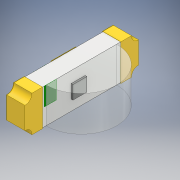
# Autodesk Inventor part: LED 3216 RA
Saved by Autodesk Inventor 2018 (Build 220112000, 112)
## iProperties
Created: 2018-02-20
Part Number: LED 3216 RA
Material: Generic
Document SubType Name: Modeling
Designer: danil
Density: 1 g/cm^3
Appearance: Generic
Author: danil
Autodesk Inventor part; units mm, degrees
ref_plane "YZ Plane" through (0, 0, 0) normal (1, 0, 0) x (0, 1, 0)
ref_plane "XZ Plane" through (0, 0, 0) normal (0, 1, 0) x (-1, 0, 0)
ref_plane "XY Plane" through (0, 0, 0) normal (0, 0, 1) x (1, 0, 0)
sketch "Sketch1" plane through (0, 0, 0) normal (0, 0, 1) x (1, 0, 0)
  arc A0 (0, -1) -> (0, 1) centre (0, 0) ccw
  line L0 (0, 0) -> (0, 1) construction
  line L1 (0, 0) -> (1, 0) construction
  line L2 (0, 0) -> (0, -1) construction
  line L3 (0, 1) -> (0, -1)
  dimension "d0" = 1
  dimension "d1" = 90
  dimension "d2" = 180
  constraints: 8 end point, 2 point on circle, 1 centre point, 1 coincident, 1 horizontal, 1 perpendicular
  measures "d0" radius of A0
  measures "d1" angle of L1 L0
  measures "d2" angle of L2 L0
extrude "Extrusion1" add sketch "Sketch1" along normal blind 1
sketch "Sketch2" plane through (0, -1, 0) normal (-1, 0, 0) x (0, 0, 1)
  line L0 (0, 2.6) -> (1, 2.6)
  line L1 (1, 2.6) -> (1, -0.6)
  line L2 (1, -0.6) -> (0, -0.6)
  line L3 (0, -0.6) -> (0, 2.6)
  line L4 (0, 2) -> (0, 0) projected
  line L5 (1, 2) -> (1, 0) projected
  arc A0 (0, 2.4) -> (0.2, 2.6) centre (0, 2.6) ccw
  arc A1 (0.8, 2.6) -> (1, 2.4) centre (1, 2.6) ccw
  arc A2 (1, -0.4) -> (0.8, -0.6) centre (1, -0.6) ccw
  arc A3 (0.2, -0.6) -> (0, -0.4) centre (0, -0.6) ccw
  point P0 (0, 1)
  point P1 (1, 1)
  point P2 (1, 1)
  dimension "d5" = 3.2
  dimension "d6" = 0.2
  constraints: 8 end point, 8 point on circle, 8 point on line, 5 coincident, 4 centre point, 3 equal radius, 2 collinear, 2 midpoint, 2 parallel, 1 horizontal, 1 perpendicular
  measures "d5" distance of L2.end L0.start
  measures "d6" radius of A0
extrude "Extrusion2" add sketch "Sketch2" along normal blind 0.5 separate body contours L0 A1 L1 A2 L2 A3 L3 A0
sketch "Sketch3" plane through (-0.5, -1, 0) normal (-1, 0, 0) x (0, 0, 1)
  line L0 (0, 2.4) -> (0, -0.4) construction
  arc A0 (0.2, -0.6) -> (0, -0.4) centre (0, -0.6) ccw projected
  line L1 (0.2, -0.6) -> (0.8, -0.6) projected
  arc A1 (1, -0.4) -> (0.8, -0.6) centre (1, -0.6) ccw projected
  line L2 (1, -0.4) -> (1, 2.4) construction
  arc A2 (0.8, 2.6) -> (1, 2.4) centre (1, 2.6) ccw projected
  line L3 (0.8, 2.6) -> (0.2, 2.6) projected
  arc A3 (0, 2.4) -> (0.2, 2.6) centre (0, 2.6) ccw projected
  line L4 (1.01, 2.4103) -> (1.01, -0.4103)
  arc A4 (1.01, -0.4103) -> (0.8103, -0.61) centre (1, -0.6) ccw
  line L5 (0.8103, -0.61) -> (0.1897, -0.61)
  arc A5 (0.1897, -0.61) -> (-0.01, -0.4103) centre (0, -0.6) ccw
  line L6 (-0.01, -0.4103) -> (-0.01, 2.4103)
  arc A6 (-0.01, 2.4103) -> (0.1897, 2.61) centre (0, 2.6) ccw
  line L7 (0.1897, 2.61) -> (0.8103, 2.61)
  arc A7 (0.8103, 2.61) -> (1.01, 2.4103) centre (1, 2.6) ccw
  line L8 (-0.01, 2.11) -> (1.01, 2.11)
  line L9 (-0.01, -0.11) -> (1.01, -0.11)
  line L10 (1.01, 1.35) -> (-0.01, 1.35)
  line L11 (-0.01, 1.35) -> (-0.01, 0.65)
  line L12 (-0.01, 0.65) -> (1.01, 0.65)
  line L13 (1.01, 0.65) -> (1.01, 1.35)
  point P0 (0, 1)
  point P1 (1.01, 1)
  point P2 (1.01, 1)
  dimension "d9" = 0.01
  dimension "d10" = 0.5
  dimension "d11" = 0.5
  dimension "d22" = 0.7
  constraints: 20 end point, 8 point on circle, 6 point on line, 4 centre point, 3 perpendicular, 2 coincident, 2 midpoint, 2 parallel, 1 horizontal, 7 other
  measures "d9" radial gap between concentric circles of A2 A7
  measures "d10" distance between parallel lines of L5 L9
  measures "d11" distance between parallel lines of L8 L7
  measures "d22" distance between parallel lines of L12 L10
extrude "Extrusion3" add sketch "Sketch3" against normal blind 0.51 separate body contours L4 L8 L6 A6 L7 A7 | L4 A4 L5 A5 L6 L9
extrude "Extrusion4" add sketch "Sketch3" along normal blind 0.01 separate body contours L4 L8 L6 A6 L7 A7 | L4 L12 L6 L10 | L4 A4 L5 A5 L6 L9
sketch "Sketch4" plane through (-0.5, -1, 0) normal (-1, 0, 0) x (0, 0, 1)
  line L0 (1, -0.4) -> (1, 2.4) projected
  line L1 (1, 0) -> (1, 2) projected
  line L2 (1, 0.098) -> (0, 0.098)
  line L3 (0, 0.098) -> (0, 0.4907)
  line L4 (0, 0.4907) -> (1, 0.4907)
  line L5 (1, 0.4907) -> (1, 0.098)
  line L6 (0, 2.4) -> (0, -0.4) projected
  point P0 (0, 1)
  point P1 (1, 1.9835)
  constraints: 8 end point, 2 parallel, 2 point on line, 1 collinear, 1 horizontal, 1 perpendicular
extrude "Extrusion5" add sketch "Sketch4" along normal blind 0.001 separate body
sketch "Sketch5" plane through (0, -1, 0) normal (1, 0, 0) x (0, 0, -1)
  line L0 (-1, -0.4) -> (-1, 2.4) projected
  line L1 (-1, -0.0582) -> (-0.4884, -0.0582)
  line L2 (-0.4884, -0.0582) -> (-0.4884, 0.2835)
  line L3 (-0.4884, 0.2835) -> (-1, 0.2835)
  line L4 (-1, 0.2835) -> (-1, -0.0582)
  constraints: 8 end point, 2 parallel, 1 horizontal, 1 perpendicular, 1 point on line
extrude "Extrusion6" add sketch "Sketch5" along normal blind 0.001 bodies 5
sketch "Sketch6" plane through (0, -1, 0) normal (1, 0, 0) x (0, 0, -1)
  line L0 (-0.6792, 0.7107) -> (-0.2977, 0.7107)
  line L1 (-0.2977, 0.7107) -> (-0.2977, 1.109)
  line L2 (-0.2977, 1.109) -> (-0.6792, 1.109)
  line L3 (-0.6792, 1.109) -> (-0.6792, 0.7107)
  point P0 (0, 1)
  constraints: 8 end point, 2 parallel, 1 horizontal, 1 perpendicular
extrude "Extrusion7" add sketch "Sketch6" along normal blind 0.05 separate body
equation "\"d11\" = d10"
body "Solid1"
body "Solid2"
body "Solid3"
body "Solid4"
body "Solid5"
body "Solid6"
